Autodesk Fusion 360 part; units mm, degrees
(part 3 of 3)
  spline S28 degree 3 poles (32.7248, 18.541) (32.6316, 18.2641) (32.4511, 17.7282) (32.036, 17.3454) (31.8353, 17.1604) knots 0 0 0 0 0.086094 0.166606 0.166606 0.166606 0.166606
  spline S29 degree 3 poles (31.8353, 17.1604) (31.5951, 17.0173) (31.0851, 16.7134) (30.4908, 16.6845) (30.1764, 16.6692) knots 0 0 0 0 0.08261 0.175377 0.175377 0.175377 0.175377
  spline S30 degree 3 poles (30.1764, 16.6692) (29.7808, 16.6955) (29.0244, 16.7456) (28.4392, 17.2241) (28.16, 17.4523) knots 0 0 0 0 0.115653 0.221163 0.221163 0.221163 0.221163
  spline S31 degree 3 poles (28.16, 17.4523) (27.9431, 17.755) (27.4744, 18.4088) (27.4359, 19.2155) (27.4151, 19.6488) knots 0 0 0 0 0.109404 0.236358 0.236358 0.236358 0.236358
  spline S32 degree 3 poles (27.4151, 19.6488) (27.4356, 20.0964) (27.4735, 20.9274) (27.9489, 21.6059) (28.1682, 21.9189) knots 0 0 0 0 0.131235 0.243597 0.243597 0.243597 0.243597
  spline S33 degree 3 poles (28.1682, 21.9189) (28.4424, 22.1544) (29.0042, 22.6369) (29.7434, 22.6962) (30.1218, 22.7265) knots 0 0 0 0 0.105595 0.216319 0.216319 0.216319 0.216319
  spline S34 degree 3 poles (30.1218, 22.7265) (30.4889, 22.6964) (31.2082, 22.6372) (31.7537, 22.166) (32.0209, 21.9353) knots 0 0 0 0 0.10743 0.210533 0.210533 0.210533 0.210533
  spline S35 degree 3 poles (32.0209, 21.9353) (32.2354, 21.6284) (32.7008, 20.9627) (32.7377, 20.148) (32.7576, 19.7088) knots 0 0 0 0 0.110094 0.23884 0.23884 0.23884 0.23884
  spline S36 degree 3 poles (32.7576, 19.7088) (32.7572, 19.6724) (32.7564, 19.5851) (32.7537, 19.4978) (32.7521, 19.4469) knots 0 0 0 0 0.010915 0.0262 0.0262 0.0262 0.0262
  line L413 (32.7521, 19.4469) -> (28.4302, 19.4469)
  spline S37 degree 3 poles (28.4302, 19.4469) (28.4585, 19.1559) (28.5109, 18.619) (28.8261, 18.1837) (28.9704, 17.9844) knots 0 0 0 0 0.08586 0.158415 0.158415 0.158415 0.158415
  spline S38 degree 3 poles (34.5475, 5.4169) (34.5677, 5.3787) (34.6088, 5.3015) (34.6804, 5.2513) (34.7166, 5.2259) knots 0 0 0 0 0.012755 0.025838 0.025838 0.025838 0.025838
  spline S39 degree 3 poles (34.7166, 5.2259) (34.7635, 5.2052) (34.8701, 5.1584) (34.9868, 5.1562) (35.0522, 5.1549) knots 0 0 0 0 0.015217 0.034603 0.034603 0.034603 0.034603
  spline S40 degree 3 poles (35.0522, 5.1549) (35.1155, 5.1572) (35.2599, 5.1623) (35.403, 5.182) (35.4834, 5.1931) knots 0 0 0 0 0.018987 0.043304 0.043304 0.043304 0.043304
  line L414 (35.4834, 5.1931) -> (35.6252, 4.3254)
  spline S41 degree 3 poles (35.6252, 4.3254) (35.4947, 4.3) (35.2494, 4.2522) (34.9998, 4.2426) (34.8831, 4.2381) knots 0 0 0 0 0.039832 0.074826 0.074826 0.074826 0.074826
  spline S42 degree 3 poles (34.8831, 4.2381) (34.7224, 4.2412) (34.4348, 4.2468) (34.1703, 4.3581) (34.0536, 4.4073) knots 0 0 0 0 0.047664 0.085336 0.085336 0.085336 0.085336
  spline S43 degree 3 poles (34.0536, 4.4073) (33.9634, 4.4665) (33.7887, 4.5812) (33.6877, 4.7638) (33.6389, 4.8521) knots 0 0 0 0 0.031834 0.061632 0.061632 0.061632 0.061632
  spline S44 degree 3 poles (33.6389, 4.8521) (33.6044, 4.9941) (33.512, 5.3741) (33.5162, 5.7661) (33.5188, 6.0117) knots 0 0 0 0 0.043707 0.116961 0.116961 0.116961 0.116961
  line L415 (33.5188, 6.0117) -> (33.5188, 9.3459)
  line L416 (33.5188, 9.3459) -> (32.7985, 9.3459)
  line L417 (32.7985, 9.3459) -> (32.7985, 10.1099)
  line L418 (32.7985, 10.1099) -> (33.5188, 10.1099)
  line L419 (33.5188, 10.1099) -> (33.5188, 11.5451)
  line L420 (33.5188, 11.5451) -> (34.4956, 12.1345)
  line L421 (34.4956, 12.1345) -> (34.4956, 10.1099)
  line L422 (34.4956, 10.1099) -> (35.4834, 10.1099)
  line L423 (35.4834, 10.1099) -> (35.4834, 9.3459)
  line L424 (35.4834, 9.3459) -> (34.4956, 9.3459)
  line L425 (34.4956, 9.3459) -> (34.4956, 5.9571)
  spline S45 degree 3 poles (34.4956, 5.9571) (34.4942, 5.8414) (34.4919, 5.659) (34.5326, 5.4817) (34.5475, 5.4169) knots 0 0 0 0 0.03454 0.054433 0.054433 0.054433 0.054433
  spline S46 degree 3 poles (18.954, 8.5328) (18.9081, 8.3627) (18.8011, 7.9667) (18.7977, 7.5558) (18.7958, 7.3214) knots 0 0 0 0 0.052651 0.122613 0.122613 0.122613 0.122613
  line L426 (18.7958, 7.3214) -> (18.7958, 4.3145)
  line L427 (18.7958, 4.3145) -> (17.8135, 4.3145)
  line L428 (17.8135, 4.3145) -> (17.8135, 10.1099)
  line L429 (17.8135, 10.1099) -> (18.6921, 10.1099)
  line L430 (18.6921, 10.1099) -> (18.6921, 9.2968)
  spline S47 degree 3 poles (18.6921, 9.2968) (18.7912, 9.4321) (18.9909, 9.705) (19.2748, 9.8889) (19.4179, 9.9817) knots 0 0 0 0 0.049853 0.100536 0.100536 0.100536 0.100536
  spline S48 degree 3 poles (19.4179, 9.9817) (19.5766, 10.0572) (19.9028, 10.2126) (20.2638, 10.2313) (20.4493, 10.2409) knots 0 0 0 0 0.052187 0.107276 0.107276 0.107276 0.107276
  spline S49 degree 3 poles (20.4493, 10.2409) (20.6485, 10.2333) (21.0203, 10.2191) (21.3514, 10.0514) (21.5052, 9.9735) knots 0 0 0 0 0.058975 0.110073 0.110073 0.110073 0.110073
  spline S50 degree 3 poles (21.5052, 9.9735) (21.6327, 9.8747) (21.8901, 9.6752) (22.0205, 9.3766) (22.0864, 9.2259) knots 0 0 0 0 0.04756 0.096056 0.096056 0.096056 0.096056
  spline S51 degree 3 poles (22.0864, 9.2259) (22.3266, 9.5218) (22.7924, 10.0955) (23.5227, 10.1934) (23.8763, 10.2409) knots 0 0 0 0 0.1098 0.212838 0.212838 0.212838 0.212838
  spline S52 degree 3 poles (23.8763, 10.2409) (24.1404, 10.2274) (24.633, 10.2023) (25.0219, 9.9024) (25.2023, 9.7634) knots 0 0 0 0 0.07719 0.143952 0.143952 0.143952 0.143952
  spline S53 degree 3 poles (25.2023, 9.7634) (25.3372, 9.5677) (25.6403, 9.1278) (25.6569, 8.5908) (25.6662, 8.2927) knots 0 0 0 0 0.069911 0.157111 0.157111 0.157111 0.157111
  line L431 (25.6662, 8.2927) -> (25.6662, 4.3145)
  line L432 (25.6662, 4.3145) -> (24.6894, 4.3145)
  line L433 (24.6894, 4.3145) -> (24.6894, 7.9653)
  spline S54 degree 3 poles (24.6894, 7.9653) (24.6893, 8.1352) (24.6893, 8.4221) (24.6215, 8.7004) (24.5939, 8.8139) knots 0 0 0 0 0.050739 0.085655 0.085655 0.085655 0.085655
  spline S55 degree 3 poles (24.5939, 8.8139) (24.5548, 8.8965) (24.475, 9.0652) (24.3242, 9.1752) (24.2473, 9.2313) knots 0 0 0 0 0.026981 0.05503 0.05503 0.05503 0.05503
  spline S56 degree 3 poles (24.2473, 9.2313) (24.1582, 9.2775) (23.9735, 9.3731) (23.7656, 9.3839) (23.658, 9.3896) knots 0 0 0 0 0.029755 0.061652 0.061652 0.061652 0.061652
  spline S57 degree 3 poles (23.658, 9.3896) (23.4642, 9.3739) (23.0834, 9.3431) (22.788, 9.1016) (22.643, 8.983) knots 0 0 0 0 0.05685 0.111677 0.111677 0.111677 0.111677
  spline S58 degree 3 poles (22.643, 8.983) (22.5256, 8.8123) (22.2582, 8.4233) (22.246, 7.9482) (22.2392, 7.6815) knots 0 0 0 0 0.060926 0.138868 0.138868 0.138868 0.138868
  line L434 (22.2392, 7.6815) -> (22.2392, 4.3145)
  line L435 (22.2392, 4.3145) -> (21.2569, 4.3145)
  line L436 (21.2569, 4.3145) -> (21.2569, 8.0799)
  spline S59 degree 3 poles (21.2569, 8.0799) (21.253, 8.2752) (21.2462, 8.622) (21.0865, 8.9283) (21.0168, 9.0621) knots 0 0 0 0 0.057612 0.102327 0.102327 0.102327 0.102327
  spline S60 degree 3 poles (21.0168, 9.0621) (20.9172, 9.1575) (20.6993, 9.3661) (20.3958, 9.3813) (20.231, 9.3896) knots 0 0 0 0 0.04006 0.087699 0.087699 0.087699 0.087699
  spline S61 degree 3 poles (20.231, 9.3896) (20.0954, 9.3805) (19.8242, 9.3623) (19.5842, 9.235) (19.4643, 9.1713) knots 0 0 0 0 0.040276 0.080523 0.080523 0.080523 0.080523
  spline S62 degree 3 poles (19.4643, 9.1713) (19.3545, 9.0886) (19.1299, 8.9196) (19.0135, 8.6636) (18.954, 8.5328) knots 0 0 0 0 0.040543 0.082899 0.082899 0.082899 0.082899
  line L437 (15.5952, 33.335) -> (14.2855, 32.0581)
  line L438 (14.2855, 32.0581) -> (14.2855, 29.2859)
  line L439 (14.2855, 29.2859) -> (13.2269, 29.2859)
  line L440 (13.2269, 29.2859) -> (13.2269, 37.2859)
  line L441 (13.2269, 37.2859) -> (14.2855, 37.2859)
  line L442 (14.2855, 37.2859) -> (14.2855, 33.3186)
  line L443 (14.2855, 33.3186) -> (18.2583, 37.2859)
  line L444 (18.2583, 37.2859) -> (19.6935, 37.2859)
  line L445 (19.6935, 37.2859) -> (16.3374, 34.0444)
  line L446 (16.3374, 34.0444) -> (19.8408, 29.2859)
  line L447 (19.8408, 29.2859) -> (18.4438, 29.2859)
  line L448 (18.4438, 29.2859) -> (15.5952, 33.335)
  spline S63 degree 3 poles (28.0427, 30.4701) (28.2157, 30.322) (28.5649, 30.0232) (29.023, 29.9829) (29.2542, 29.9626) knots 0 0 0 0 0.066533 0.134307 0.134307 0.134307 0.134307
  spline S64 degree 3 poles (29.2542, 29.9626) (29.4253, 29.9727) (29.7563, 29.9922) (30.0396, 30.1636) (30.1764, 30.2463) knots 0 0 0 0 0.050568 0.097792 0.097792 0.097792 0.097792
  spline S65 degree 3 poles (30.1764, 30.2463) (30.2998, 30.3628) (30.5699, 30.6178) (30.7074, 30.964) (30.7821, 31.1522) knots 0 0 0 0 0.050293 0.110147 0.110147 0.110147 0.110147
  line L449 (30.7821, 31.1522) -> (31.7971, 31.0267)
  spline S66 degree 3 poles (31.7971, 31.0267) (31.7039, 30.7497) (31.5234, 30.2138) (31.1083, 29.831) (30.9076, 29.646) knots 0 0 0 0 0.086093 0.166606 0.166606 0.166606 0.166606
  spline S67 degree 3 poles (30.9076, 29.646) (30.6674, 29.5029) (30.1574, 29.1991) (29.5631, 29.1702) (29.2487, 29.1549) knots 0 0 0 0 0.082609 0.175376 0.175376 0.175376 0.175376
  spline S68 degree 3 poles (29.2487, 29.1549) (28.8532, 29.1811) (28.0967, 29.2313) (27.5115, 29.7097) (27.2323, 29.938) knots 0 0 0 0 0.115653 0.221163 0.221163 0.221163 0.221163
  spline S69 degree 3 poles (27.2323, 29.938) (27.0154, 30.2406) (26.5467, 30.8944) (26.5082, 31.7011) (26.4874, 32.1345) knots 0 0 0 0 0.109405 0.236358 0.236358 0.236358 0.236358
  spline S70 degree 3 poles (26.4874, 32.1345) (26.5079, 32.5821) (26.5458, 33.4131) (27.0212, 34.0916) (27.2405, 34.4046) knots 0 0 0 0 0.131235 0.243597 0.243597 0.243597 0.243597
  spline S71 degree 3 poles (27.2405, 34.4046) (27.5147, 34.6401) (28.0765, 35.1226) (28.8157, 35.1819) (29.1941, 35.2122) knots 0 0 0 0 0.105595 0.216319 0.216319 0.216319 0.216319
  spline S72 degree 3 poles (29.1941, 35.2122) (29.5612, 35.182) (30.2806, 35.1229) (30.826, 34.6517) (31.0932, 34.4209) knots 0 0 0 0 0.10743 0.210533 0.210533 0.210533 0.210533
  spline S73 degree 3 poles (31.0932, 34.4209) (31.3077, 34.1141) (31.7731, 33.4484) (31.81, 32.6336) (31.8299, 32.1945) knots 0 0 0 0 0.110094 0.238839 0.238839 0.238839 0.238839
  spline S74 degree 3 poles (31.8299, 32.1945) (31.8295, 32.1581) (31.8287, 32.0708) (31.826, 31.9835) (31.8244, 31.9325) knots 0 0 0 0 0.010915 0.0262 0.0262 0.0262 0.0262
  line L450 (31.8244, 31.9325) -> (27.5025, 31.9325)
  spline S75 degree 3 poles (27.5025, 31.9325) (27.5308, 31.6416) (27.5832, 31.1047) (27.8984, 30.6694) (28.0427, 30.4701) knots 0 0 0 0 0.08586 0.158415 0.158415 0.158415 0.158415
  line L451 (11.5652, 5.2586) -> (16.4765, 5.2586)
  line L452 (16.4765, 5.2586) -> (16.4765, 4.3145)
  line L453 (16.4765, 4.3145) -> (10.5065, 4.3145)
  line L454 (10.5065, 4.3145) -> (10.5065, 12.3145)
  line L455 (10.5065, 12.3145) -> (16.291, 12.3145)
  line L456 (16.291, 12.3145) -> (16.291, 11.3705)
  line L457 (16.291, 11.3705) -> (11.5652, 11.3705)
  line L458 (11.5652, 11.3705) -> (11.5652, 8.9203)
  line L459 (11.5652, 8.9203) -> (15.9909, 8.9203)
  line L460 (15.9909, 8.9203) -> (15.9909, 7.9817)
  line L461 (15.9909, 7.9817) -> (11.5652, 7.9817)
  line L462 (11.5652, 7.9817) -> (11.5652, 5.2586)
  spline S76 degree 3 poles (38.4411, 2.9012) (38.3557, 2.7537) (38.1975, 2.4803) (37.9533, 2.2809) (37.8408, 2.189) knots 0 0 0 0 0.050608 0.093822 0.093822 0.093822 0.093822
  spline S77 degree 3 poles (37.8408, 2.189) (37.7198, 2.123) (37.4683, 1.9857) (37.1818, 1.9705) (37.0332, 1.9626) knots 0 0 0 0 0.04081 0.084832 0.084832 0.084832 0.084832
  spline S78 degree 3 poles (37.0332, 1.9626) (36.9324, 1.9688) (36.7165, 1.9821) (36.5102, 2.0476) (36.4001, 2.0826) knots 0 0 0 0 0.030163 0.064648 0.064648 0.064648 0.064648
  line L463 (36.4001, 2.0826) -> (36.291, 3.0048)
  spline S79 degree 3 poles (36.291, 3.0048) (36.391, 2.9794) (36.5756, 2.9325) (36.7658, 2.9222) (36.8531, 2.9175) knots 0 0 0 0 0.030853 0.057001 0.057001 0.057001 0.057001
  spline S80 degree 3 poles (36.8531, 2.9175) (36.9528, 2.92) (37.1344, 2.9246) (37.3015, 2.9949) (37.3769, 3.0267) knots 0 0 0 0 0.029594 0.053932 0.053932 0.053932 0.053932
  spline S81 degree 3 poles (37.3769, 3.0267) (37.4397, 3.067) (37.5663, 3.1484) (37.6544, 3.2706) (37.6989, 3.3323) knots 0 0 0 0 0.022157 0.044743 0.044743 0.044743 0.044743
  spline S82 degree 3 poles (37.6989, 3.3323) (37.7407, 3.4172) (37.8571, 3.654) (37.9436, 3.9035) (37.999, 4.0635) knots 0 0 0 0 0.028377 0.079105 0.079105 0.079105 0.079105
  spline S83 degree 3 poles (37.999, 4.0635) (38.0107, 4.0972) (38.0387, 4.1777) (38.0688, 4.2573) (38.0864, 4.3036) knots 0 0 0 0 0.0107 0.02555 0.02555 0.02555 0.02555
  line L464 (38.0864, 4.3036) -> (35.8872, 10.1099)
  line L465 (35.8872, 10.1099) -> (36.9458, 10.1099)
  line L466 (36.9458, 10.1099) -> (38.1518, 6.7538)
  spline S84 degree 3 poles (38.1518, 6.7538) (38.2285, 6.5363) (38.3845, 6.0939) (38.5088, 5.6414) (38.572, 5.4114) knots 0 0 0 0 0.069157 0.140705 0.140705 0.140705 0.140705
  spline S85 degree 3 poles (38.572, 5.4114) (38.631, 5.6351) (38.7483, 6.0806) (38.9002, 6.5155) (38.9759, 6.732) knots 0 0 0 0 0.069376 0.138143 0.138143 0.138143 0.138143
  line L467 (38.9759, 6.732) -> (40.2146, 10.1099)
  line L468 (40.2146, 10.1099) -> (41.1969, 10.1099)
  line L469 (41.1969, 10.1099) -> (38.9922, 4.2163)
  spline S86 degree 3 poles (38.9922, 4.2163) (38.8921, 3.9454) (38.7272, 3.499) (38.5218, 3.0699) (38.4411, 2.9012) knots 0 0 0 0 0.086568 0.142661 0.142661 0.142661 0.142661
  line L470 (0, 41.4903) -> (2.5, 41.4903)
  line L471 (2.5, 41.4903) -> (2.5, 36.4903)
  line L472 (2.5, 36.4903) -> (0, 36.4903)
  line L473 (0, 36.4903) -> (0, 31.4903)
  line L474 (0, 31.4903) -> (2.5, 31.4903)
  line L475 (2.5, 31.4903) -> (2.5, 26.4903)
  line L476 (2.5, 26.4903) -> (0, 26.4903)
  line L477 (0, 26.4903) -> (0, 21.4903)
  line L478 (0, 21.4903) -> (2.5, 21.4903)
  line L479 (2.5, 21.4903) -> (2.5, 16.4903)
  line L480 (2.5, 16.4903) -> (0, 16.4903)
  line L481 (0, 16.4903) -> (0, 11.4903)
  line L482 (0, 11.4903) -> (2.5, 11.4903)
  line L483 (2.5, 11.4903) -> (2.5, 6.4903)
  line L484 (2.5, 6.4903) -> (0, 6.4903)
  line L485 (0, 6.4903) -> (0, -3.5097)
  line L486 (0, -3.5097) -> (2.5, -3.5097)
  line L487 (2.5, -3.5097) -> (2.5, -1.0097)
  line L488 (2.5, -1.0097) -> (7.5, -1.0097)
  line L489 (7.5, -1.0097) -> (7.5, -3.5097)
  line L490 (7.5, -3.5097) -> (12.5, -3.5097)
  line L491 (12.5, -3.5097) -> (12.5, -1.0097)
  line L492 (12.5, -1.0097) -> (17.5, -1.0097)
  line L493 (17.5, -1.0097) -> (17.5, -3.5097)
  line L494 (17.5, -3.5097) -> (22.5, -3.5097)
  line L495 (22.5, -3.5097) -> (22.5, -1.0097)
  line L496 (22.5, -1.0097) -> (27.5, -1.0097)
  line L497 (27.5, -1.0097) -> (27.5, -3.5097)
  line L498 (27.5, -3.5097) -> (32.5, -3.5097)
  line L499 (32.5, -3.5097) -> (32.5, -1.0097)
  line L500 (32.5, -1.0097) -> (37.5, -1.0097)
  line L501 (37.5, -1.0097) -> (37.5, -3.5097)
  line L502 (37.5, -3.5097) -> (42.5, -3.5097)
  line L503 (42.5, -3.5097) -> (42.5, -1.0097)
  line L504 (42.5, -1.0097) -> (47.5, -1.0097)
  line L505 (47.5, -1.0097) -> (47.5, -3.5097)
  line L506 (47.5, -3.5097) -> (50, -3.5097)
  line L507 (50, -3.5097) -> (50, 6.4903)
  line L508 (50, 6.4903) -> (47.5, 6.4903)
  line L509 (47.5, 6.4903) -> (47.5, 11.4903)
  line L510 (47.5, 11.4903) -> (50, 11.4903)
  line L511 (50, 11.4903) -> (50, 16.4903)
  line L512 (50, 16.4903) -> (47.5, 16.4903)
  line L513 (47.5, 16.4903) -> (47.5, 21.4903)
  line L514 (47.5, 21.4903) -> (50, 21.4903)
  line L515 (50, 21.4903) -> (50, 26.4903)
  line L516 (50, 26.4903) -> (47.5, 26.4903)
  line L517 (47.5, 26.4903) -> (47.5, 31.4903)
  line L518 (47.5, 31.4903) -> (50, 31.4903)
  line L519 (50, 31.4903) -> (50, 36.4903)
  line L520 (50, 36.4903) -> (47.5, 36.4903)
  line L521 (47.5, 36.4903) -> (47.5, 41.4903)
  line L522 (47.5, 41.4903) -> (50, 41.4903)
  line L523 (50, 41.4903) -> (50, 46.4903)
  line L524 (50, 46.4903) -> (47.3, 46.4903)
  line L525 (47.3, 46.4903) -> (47.3, 43.9903)
  line L526 (47.3, 43.9903) -> (42.7, 43.9903)
  line L527 (42.7, 43.9903) -> (42.7, 46.4903)
  line L528 (42.7, 46.4903) -> (37.3, 46.4903)
  line L529 (37.3, 46.4903) -> (37.3, 43.9903)
  line L530 (37.3, 43.9903) -> (32.7, 43.9903)
  line L531 (32.7, 43.9903) -> (32.7, 46.4903)
  line L532 (32.7, 46.4903) -> (27.3, 46.4903)
  line L533 (27.3, 46.4903) -> (27.3, 43.9903)
  line L534 (27.3, 43.9903) -> (22.7, 43.9903)
  line L535 (22.7, 43.9903) -> (22.7, 46.4903)
  line L536 (22.7, 46.4903) -> (17.3, 46.4903)
  line L537 (17.3, 46.4903) -> (17.3, 43.9903)
  line L538 (17.3, 43.9903) -> (12.7, 43.9903)
  line L539 (12.7, 43.9903) -> (12.7, 46.4903)
  line L540 (12.7, 46.4903) -> (7.3, 46.4903)
  line L541 (7.3, 46.4903) -> (7.3, 43.9903)
  line L542 (7.3, 43.9903) -> (2.7, 43.9903)
  line L543 (2.7, 43.9903) -> (2.7, 46.4903)
  line L544 (2.7, 46.4903) -> (0, 46.4903)
  line L545 (0, 46.4903) -> (0, 41.4903)
  spline S87 degree 3 poles (34.6539, 29.3623) (34.5306, 29.4347) (34.2897, 29.5762) (34.1036, 29.7844) (34.0127, 29.8862) knots 0 0 0 0 0.042587 0.083249 0.083249 0.083249 0.083249
  line L546 (34.0127, 29.8862) -> (34.0127, 27.0649)
  line L547 (34.0127, 27.0649) -> (33.0304, 27.0649)
  line L548 (33.0304, 27.0649) -> (33.0304, 35.0812)
  line L549 (33.0304, 35.0812) -> (33.9254, 35.0812)
  line L550 (33.9254, 35.0812) -> (33.9254, 34.3282)
  spline S88 degree 3 poles (33.9254, 34.3282) (34.031, 34.4644) (34.2329, 34.725) (34.5087, 34.9052) (34.6402, 34.9912) knots 0 0 0 0 0.051297 0.098108 0.098108 0.098108 0.098108
  spline S89 degree 3 poles (34.6402, 34.9912) (34.785, 35.0556) (35.092, 35.1923) (35.4283, 35.2053) (35.6061, 35.2122) knots 0 0 0 0 0.04708 0.099893 0.099893 0.099893 0.099893
  spline S90 degree 3 poles (35.6061, 35.2122) (35.8441, 35.1977) (36.3099, 35.1694) (36.7168, 34.9416) (36.9158, 34.8302) knots 0 0 0 0 0.0705 0.138 0.138 0.138 0.138
  spline S91 degree 3 poles (36.9158, 34.8302) (37.0946, 34.687) (37.4615, 34.3929) (37.6671, 33.9696) (37.7726, 33.7525) knots 0 0 0 0 0.06782 0.139223 0.139223 0.139223 0.139223
  spline S92 degree 3 poles (37.7726, 33.7525) (37.8569, 33.5117) (38.0299, 33.018) (38.051, 32.4951) (38.0618, 32.2272) knots 0 0 0 0 0.076077 0.15601 0.15601 0.15601 0.15601
  spline S93 degree 3 poles (38.0618, 32.2272) (38.0504, 31.9424) (38.0283, 31.3914) (37.8356, 30.875) (37.7426, 30.6256) knots 0 0 0 0 0.084892 0.164238 0.164238 0.164238 0.164238
  spline S94 degree 3 poles (37.7426, 30.6256) (37.6265, 30.4036) (37.3995, 29.9694) (37.0068, 29.677) (36.8149, 29.5342) knots 0 0 0 0 0.074084 0.14489 0.14489 0.14489 0.14489
  spline S95 degree 3 poles (36.8149, 29.5342) (36.6115, 29.4236) (36.2116, 29.2062) (35.758, 29.1718) (35.5352, 29.1549) knots 0 0 0 0 0.068591 0.134825 0.134825 0.134825 0.134825
  spline S96 degree 3 poles (35.5352, 29.1549) (35.3776, 29.1626) (35.0709, 29.1774) (34.7903, 29.3018) (34.6539, 29.3623) knots 0 0 0 0 0.046877 0.091234 0.091234 0.091234 0.091234
  line L551 (22.9786, 35.2122) -> (23.3457, 35.182)
  line L552 (23.3457, 35.182) -> (24.065, 35.1229)
  line L553 (24.065, 35.1229) -> (24.6105, 34.6517)
  line L554 (24.6105, 34.6517) -> (24.8776, 34.4209)
  line L555 (24.6921, 29.646) -> (24.4518, 29.5029)
  line L556 (24.4518, 29.5029) -> (23.9418, 29.1991)
  line L557 (23.9418, 29.1991) -> (23.3475, 29.1702)
  line L558 (23.3475, 29.1702) -> (23.0332, 29.1549)
  line L559 (27.2323, 29.938) -> (27.0154, 30.2406)
  line L560 (27.0154, 30.2406) -> (26.5467, 30.8944)
  line L561 (26.5467, 30.8944) -> (26.5082, 31.7011)
  line L562 (26.5082, 31.7011) -> (26.4874, 32.1345)
  line L563 (23.0332, 29.1549) -> (22.6376, 29.1811)
  line L564 (22.6376, 29.1811) -> (21.8812, 29.2313)
  line L565 (21.8812, 29.2313) -> (21.296, 29.7097)
  line L566 (21.296, 29.7097) -> (21.0168, 29.938)
  line L567 (25.6143, 32.1945) -> (25.614, 32.1581)
  line L568 (25.614, 32.1581) -> (25.6131, 32.0708)
  line L569 (25.6131, 32.0708) -> (25.6104, 31.9835)
  line L570 (25.6104, 31.9835) -> (25.6089, 31.9325)
  line L571 (24.8776, 34.4209) -> (25.0922, 34.1141)
  line L572 (25.0922, 34.1141) -> (25.5575, 33.4484)
  line L573 (25.5575, 33.4484) -> (25.5944, 32.6336)
  line L574 (25.5944, 32.6336) -> (25.6143, 32.1945)
  line L575 (21.0168, 29.938) -> (20.7998, 30.2406)
  line L576 (20.7998, 30.2406) -> (20.3312, 30.8944)
  line L577 (20.3312, 30.8944) -> (20.2926, 31.7011)
  line L578 (20.2926, 31.7011) -> (20.2719, 32.1345)
  line L579 (34.6402, 34.9912) -> (34.785, 35.0556)
  line L580 (34.785, 35.0556) -> (35.092, 35.1923)
  line L581 (35.092, 35.1923) -> (35.4283, 35.2053)
  line L582 (35.4283, 35.2053) -> (35.6061, 35.2122)
  line L583 (35.6252, 4.3254) -> (35.4947, 4.3)
  line L584 (35.4947, 4.3) -> (35.2494, 4.2522)
  line L585 (35.2494, 4.2522) -> (34.9998, 4.2426)
  line L586 (34.9998, 4.2426) -> (34.8831, 4.2381)
  line L587 (35.5352, 29.1549) -> (35.3776, 29.1626)
  line L588 (35.3776, 29.1626) -> (35.0709, 29.1774)
  line L589 (35.0709, 29.1774) -> (34.7903, 29.3018)
  line L590 (34.7903, 29.3018) -> (34.6539, 29.3623)
  line L591 (37.8408, 2.189) -> (37.7198, 2.123)
  line L592 (37.7198, 2.123) -> (37.4683, 1.9857)
  line L593 (37.4683, 1.9857) -> (37.1818, 1.9705)
  line L594 (37.1818, 1.9705) -> (37.0332, 1.9626)
  line L595 (37.7426, 30.6256) -> (37.6265, 30.4036)
  line L596 (37.6265, 30.4036) -> (37.3995, 29.9694)
  line L597 (37.3995, 29.9694) -> (37.0068, 29.677)
  line L598 (37.0068, 29.677) -> (36.8149, 29.5342)
  line L599 (34.7166, 5.2259) -> (34.7635, 5.2052)
  line L600 (34.7635, 5.2052) -> (34.8701, 5.1584)
  line L601 (34.8701, 5.1584) -> (34.9868, 5.1562)
  line L602 (34.9868, 5.1562) -> (35.0522, 5.1549)
  line L603 (36.8531, 2.9175) -> (36.9528, 2.92)
  line L604 (36.9528, 2.92) -> (37.1344, 2.9246)
  line L605 (37.1344, 2.9246) -> (37.3015, 2.9949)
  line L606 (37.3015, 2.9949) -> (37.3769, 3.0267)
  line L607 (30.1764, 16.6692) -> (29.7808, 16.6955)
  line L608 (29.7808, 16.6955) -> (29.0244, 16.7456)
  line L609 (29.0244, 16.7456) -> (28.4392, 17.2241)
  line L610 (28.4392, 17.2241) -> (28.16, 17.4523)
  line L611 (28.1682, 21.9189) -> (28.4424, 22.1544)
  line L612 (28.4424, 22.1544) -> (29.0042, 22.6369)
  line L613 (29.0042, 22.6369) -> (29.7434, 22.6962)
  line L614 (29.7434, 22.6962) -> (30.1218, 22.7265)
  line L615 (35.0522, 5.1549) -> (35.1155, 5.1572)
  line L616 (35.1155, 5.1572) -> (35.2599, 5.1623)
  line L617 (35.2599, 5.1623) -> (35.403, 5.182)
  line L618 (35.403, 5.182) -> (35.4834, 5.1931)
  line L619 (38.4411, 2.9012) -> (38.3557, 2.7537)
  line L620 (38.3557, 2.7537) -> (38.1975, 2.4803)
  line L621 (38.1975, 2.4803) -> (37.9533, 2.2809)
  line L622 (37.9533, 2.2809) -> (37.8408, 2.189)
  line L623 (31.8353, 17.1604) -> (31.5951, 17.0173)
  line L624 (31.5951, 17.0173) -> (31.0851, 16.7134)
  line L625 (31.0851, 16.7134) -> (30.4908, 16.6845)
  line L626 (30.4908, 16.6845) -> (30.1764, 16.6692)
  line L627 (36.291, 3.0048) -> (36.391, 2.9794)
  line L628 (36.391, 2.9794) -> (36.5756, 2.9325)
  line L629 (36.5756, 2.9325) -> (36.7658, 2.9222)
  line L630 (36.7658, 2.9222) -> (36.8531, 2.9175)
  line L631 (37.0332, 1.9626) -> (36.9324, 1.9688)
  line L632 (36.9324, 1.9688) -> (36.7165, 1.9821)
  line L633 (36.7165, 1.9821) -> (36.5102, 2.0476)
  line L634 (36.5102, 2.0476) -> (36.4001, 2.0826)
  line L635 (34.4956, 5.9571) -> (34.4942, 5.8414)
  line L636 (34.4942, 5.8414) -> (34.4919, 5.659)
  line L637 (34.4919, 5.659) -> (34.5326, 5.4817)
  line L638 (34.5326, 5.4817) -> (34.5475, 5.4169)
  line L639 (27.4151, 19.6488) -> (27.4356, 20.0964)
  line L640 (27.4356, 20.0964) -> (27.4735, 20.9274)
  line L641 (27.4735, 20.9274) -> (27.9489, 21.6059)
  line L642 (27.9489, 21.6059) -> (28.1682, 21.9189)
  line L643 (38.9922, 4.2163) -> (38.8921, 3.9454)
  line L644 (38.8921, 3.9454) -> (38.7272, 3.499)
  line L645 (38.7272, 3.499) -> (38.5218, 3.0699)
  line L646 (38.5218, 3.0699) -> (38.4411, 2.9012)
  line L647 (37.7726, 33.7525) -> (37.8569, 33.5117)
  line L648 (37.8569, 33.5117) -> (38.0299, 33.018)
  line L649 (38.0299, 33.018) -> (38.051, 32.4951)
  line L650 (38.051, 32.4951) -> (38.0618, 32.2272)
  line L651 (37.6989, 3.3323) -> (37.7407, 3.4172)
  line L652 (37.7407, 3.4172) -> (37.8571, 3.654)
  line L653 (37.8571, 3.654) -> (37.9436, 3.9035)
  line L654 (37.9436, 3.9035) -> (37.999, 4.0635)
  line L655 (32.7248, 18.541) -> (32.6316, 18.2641)
  line L656 (32.6316, 18.2641) -> (32.4511, 17.7282)
  line L657 (32.4511, 17.7282) -> (32.036, 17.3454)
  line L658 (32.036, 17.3454) -> (31.8353, 17.1604)
  line L659 (36.9158, 34.8302) -> (37.0946, 34.687)
  line L660 (37.0946, 34.687) -> (37.4615, 34.3929)
  line L661 (37.4615, 34.3929) -> (37.6671, 33.9696)
  line L662 (37.6671, 33.9696) -> (37.7726, 33.7525)
  line L663 (34.6539, 29.3623) -> (34.5306, 29.4347)
  line L664 (34.5306, 29.4347) -> (34.2897, 29.5762)
  line L665 (34.2897, 29.5762) -> (34.1036, 29.7844)
  line L666 (34.1036, 29.7844) -> (34.0127, 29.8862)
  line L667 (20.2719, 32.1345) -> (20.2923, 32.5821)
  line L668 (20.2923, 32.5821) -> (20.3302, 33.4131)
  line L669 (20.3302, 33.4131) -> (20.8057, 34.0916)
  line L670 (20.8057, 34.0916) -> (21.025, 34.4046)
  line L671 (21.2869, 31.9325) -> (21.3153, 31.6416)
  line L672 (21.3153, 31.6416) -> (21.3677, 31.1047)
  line L673 (21.3677, 31.1047) -> (21.6828, 30.6694)
  line L674 (21.6828, 30.6694) -> (21.8271, 30.4701)
  line L675 (25.5816, 31.0267) -> (25.4883, 30.7497)
  line L676 (25.4883, 30.7497) -> (25.3079, 30.2138)
  line L677 (25.3079, 30.2138) -> (24.8927, 29.831)
  line L678 (24.8927, 29.831) -> (24.6921, 29.646)
  line L679 (23.9608, 30.2463) -> (24.0842, 30.3628)
  line L680 (24.0842, 30.3628) -> (24.3544, 30.6178)
  line L681 (24.3544, 30.6178) -> (24.4919, 30.964)
  line L682 (24.4919, 30.964) -> (24.5666, 31.1522)
  line L683 (23.0386, 29.9626) -> (23.2097, 29.9727)
  line L684 (23.2097, 29.9727) -> (23.5407, 29.9922)
  line L685 (23.5407, 29.9922) -> (23.824, 30.1636)
  line L686 (23.824, 30.1636) -> (23.9608, 30.2463)
  line L687 (26.4874, 32.1345) -> (26.5079, 32.5821)
  line L688 (26.5079, 32.5821) -> (26.5458, 33.4131)
  line L689 (26.5458, 33.4131) -> (27.0212, 34.0916)
  line L690 (27.0212, 34.0916) -> (27.2405, 34.4046)
  line L691 (21.8271, 30.4701) -> (22.0001, 30.322)
  line L692 (22.0001, 30.322) -> (22.3494, 30.0232)
  line L693 (22.3494, 30.0232) -> (22.8074, 29.9829)
  line L694 (22.8074, 29.9829) -> (23.0386, 29.9626)
  line L695 (21.025, 34.4046) -> (21.2992, 34.6401)
  line L696 (21.2992, 34.6401) -> (21.8609, 35.1226)
  line L697 (21.8609, 35.1226) -> (22.6002, 35.1819)
  line L698 (22.6002, 35.1819) -> (22.9786, 35.2122)
  line L699 (31.0932, 34.4209) -> (31.3077, 34.1141)
  line L700 (31.3077, 34.1141) -> (31.7731, 33.4484)
  line L701 (31.7731, 33.4484) -> (31.81, 32.6336)
  line L702 (31.81, 32.6336) -> (31.8299, 32.1945)
  line L703 (31.0086, 9.8589) -> (31.1873, 9.7156)
  line L704 (31.1873, 9.7156) -> (31.5543, 9.4215)
  line L705 (31.5543, 9.4215) -> (31.7599, 8.9982)
  line L706 (31.7599, 8.9982) -> (31.8653, 8.7811)
  line L707 (30.9076, 29.646) -> (30.6674, 29.5029)
  line L708 (30.6674, 29.5029) -> (30.1574, 29.1991)
  line L709 (30.1574, 29.1991) -> (29.5631, 29.1702)
  line L710 (29.5631, 29.1702) -> (29.2487, 29.1549)
  line L711 (31.8653, 8.7811) -> (31.9497, 8.5404)
  line L712 (31.9497, 8.5404) -> (32.1226, 8.0467)
  line L713 (32.1226, 8.0467) -> (32.1438, 7.5238)
  line L714 (32.1438, 7.5238) -> (32.1546, 7.2559)
  line L715 (28.0427, 30.4701) -> (28.2157, 30.322)
  line L716 (28.2157, 30.322) -> (28.5649, 30.0232)
  line L717 (28.5649, 30.0232) -> (29.023, 29.9829)
  line L718 (29.023, 29.9829) -> (29.2542, 29.9626)
  line L719 (23.658, 9.3896) -> (23.4642, 9.3739)
  line L720 (23.4642, 9.3739) -> (23.0834, 9.3431)
  line L721 (23.0834, 9.3431) -> (22.788, 9.1016)
  line L722 (22.788, 9.1016) -> (22.643, 8.983)
  line L723 (32.7576, 19.7088) -> (32.7572, 19.6724)
  line L724 (32.7572, 19.6724) -> (32.7564, 19.5851)
  line L725 (32.7564, 19.5851) -> (32.7537, 19.4978)
  line L726 (32.7537, 19.4978) -> (32.7521, 19.4469)
  line L727 (27.5025, 31.9325) -> (27.5308, 31.6416)
  line L728 (27.5308, 31.6416) -> (27.5832, 31.1047)
  line L729 (27.5832, 31.1047) -> (27.8984, 30.6694)
  line L730 (27.8984, 30.6694) -> (28.0427, 30.4701)
  line L731 (18.6921, 9.2968) -> (18.7912, 9.4321)
  line L732 (18.7912, 9.4321) -> (18.9909, 9.705)
  line L733 (18.9909, 9.705) -> (19.2748, 9.8889)
  line L734 (19.2748, 9.8889) -> (19.4179, 9.9817)
  line L735 (28.16, 17.4523) -> (27.9431, 17.755)
  line L736 (27.9431, 17.755) -> (27.4744, 18.4088)
  line L737 (27.4744, 18.4088) -> (27.4359, 19.2155)
  line L738 (27.4359, 19.2155) -> (27.4151, 19.6488)
  line L739 (30.1764, 30.2463) -> (30.2998, 30.3628)
  line L740 (30.2998, 30.3628) -> (30.5699, 30.6178)
  line L741 (30.5699, 30.6178) -> (30.7074, 30.964)
  line L742 (30.7074, 30.964) -> (30.7821, 31.1522)
  line L743 (33.6389, 4.8521) -> (33.6044, 4.9941)
  line L744 (33.6044, 4.9941) -> (33.512, 5.3741)
  line L745 (33.512, 5.3741) -> (33.5162, 5.7661)
  line L746 (33.5162, 5.7661) -> (33.5188, 6.0117)
  line L747 (22.0864, 9.2259) -> (22.3266, 9.5218)
  line L748 (22.3266, 9.5218) -> (22.7924, 10.0955)
  line L749 (22.7924, 10.0955) -> (23.5227, 10.1934)
  line L750 (23.5227, 10.1934) -> (23.8763, 10.2409)
  line L751 (29.628, 4.1836) -> (29.4704, 4.1912)
  line L752 (29.4704, 4.1912) -> (29.1636, 4.2061)
  line L753 (29.1636, 4.2061) -> (28.8831, 4.3305)
  line L754 (28.8831, 4.3305) -> (28.7467, 4.3909)
  line L755 (29.6989, 10.2409) -> (29.9369, 10.2264)
  line L756 (29.9369, 10.2264) -> (30.4026, 10.198)
  line L757 (30.4026, 10.198) -> (30.8096, 9.9703)
  line L758 (30.8096, 9.9703) -> (31.0086, 9.8589)
  line L759 (22.3947, 17.9516) -> (22.4524, 18.1314)
  line L760 (22.4524, 18.1314) -> (22.5902, 18.5603)
  line L761 (22.5902, 18.5603) -> (22.7358, 18.9865)
  line L762 (22.7358, 18.9865) -> (22.8203, 19.234)
  line L763 (28.733, 10.0199) -> (28.8777, 10.0843)
  line L764 (28.8777, 10.0843) -> (29.1848, 10.2209)
  line L765 (29.1848, 10.2209) -> (29.5211, 10.234)
  line L766 (29.5211, 10.234) -> (29.6989, 10.2409)
  line L767 (29.1941, 35.2122) -> (29.5612, 35.182)
  line L768 (29.5612, 35.182) -> (30.2806, 35.1229)
  line L769 (30.2806, 35.1229) -> (30.826, 34.6517)
  line L770 (30.826, 34.6517) -> (31.0932, 34.4209)
  line L771 (19.4643, 9.1713) -> (19.3545, 9.0886)
  line L772 (19.3545, 9.0886) -> (19.1299, 8.9196)
  line L773 (19.1299, 8.9196) -> (19.0135, 8.6636)
  line L774 (19.0135, 8.6636) -> (18.954, 8.5328)
  line L775 (38.1518, 6.7538) -> (38.2285, 6.5363)
  line L776 (38.2285, 6.5363) -> (38.3845, 6.0939)
  line L777 (38.3845, 6.0939) -> (38.5088, 5.6414)
  line L778 (38.5088, 5.6414) -> (38.572, 5.4114)
  line L779 (28.7467, 4.3909) -> (28.6234, 4.4633)
  line L780 (28.6234, 4.4633) -> (28.3825, 4.6049)
  line L781 (28.3825, 4.6049) -> (28.1964, 4.8131)
  line L782 (28.1964, 4.8131) -> (28.1055, 4.9148)
  line L783 (32.0209, 21.9353) -> (32.2354, 21.6284)
  line L784 (32.2354, 21.6284) -> (32.7008, 20.9627)
  line L785 (32.7008, 20.9627) -> (32.7377, 20.148)
  line L786 (32.7377, 20.148) -> (32.7576, 19.7088)
  line L787 (20.4493, 10.2409) -> (20.6485, 10.2333)
  line L788 (20.6485, 10.2333) -> (21.0203, 10.2191)
  line L789 (21.0203, 10.2191) -> (21.3514, 10.0514)
  line L790 (21.3514, 10.0514) -> (21.5052, 9.9735)
  line L791 (31.8299, 32.1945) -> (31.8295, 32.1581)
  line L792 (31.8295, 32.1581) -> (31.8287, 32.0708)
  line L793 (31.8287, 32.0708) -> (31.826, 31.9835)
  line L794 (31.826, 31.9835) -> (31.8244, 31.9325)
  line L795 (18.954, 8.5328) -> (18.9081, 8.3627)
  line L796 (18.9081, 8.3627) -> (18.8011, 7.9667)
  line L797 (18.8011, 7.9667) -> (18.7977, 7.5558)
  line L798 (18.7977, 7.5558) -> (18.7958, 7.3214)
  line L799 (34.5475, 5.4169) -> (34.5677, 5.3787)
  line L800 (34.5677, 5.3787) -> (34.6088, 5.3015)
  line L801 (34.6088, 5.3015) -> (34.6804, 5.2513)
  line L802 (34.6804, 5.2513) -> (34.7166, 5.2259)
  line L803 (28.4302, 19.4469) -> (28.4585, 19.1559)
  line L804 (28.4585, 19.1559) -> (28.5109, 18.619)
  line L805 (28.5109, 18.619) -> (28.8261, 18.1837)
  line L806 (28.8261, 18.1837) -> (28.9704, 17.9844)
  line L807 (31.8353, 5.6542) -> (31.7193, 5.4322)
  line L808 (31.7193, 5.4322) -> (31.4922, 4.9981)
  line L809 (31.4922, 4.9981) -> (31.0995, 4.7057)
  line L810 (31.0995, 4.7057) -> (30.9076, 4.5628)
  line L811 (33.9254, 34.3282) -> (34.031, 34.4644)
  line L812 (34.031, 34.4644) -> (34.2329, 34.725)
  line L813 (34.2329, 34.725) -> (34.5087, 34.9052)
  line L814 (34.5087, 34.9052) -> (34.6402, 34.9912)
  line L815 (32.1546, 7.2559) -> (32.1432, 6.9711)
  line L816 (32.1432, 6.9711) -> (32.1211, 6.4201)
  line L817 (32.1211, 6.4201) -> (31.9284, 5.9037)
  line L818 (31.9284, 5.9037) -> (31.8353, 5.6542)
  line L819 (38.0618, 32.2272) -> (38.0504, 31.9424)
  line L820 (38.0504, 31.9424) -> (38.0283, 31.3914)
  line L821 (38.0283, 31.3914) -> (37.8356, 30.875)
  line L822 (37.8356, 30.875) -> (37.7426, 30.6256)
  line L823 (29.2542, 29.9626) -> (29.4253, 29.9727)
  line L824 (29.4253, 29.9727) -> (29.7563, 29.9922)
  line L825 (29.7563, 29.9922) -> (30.0396, 30.1636)
  line L826 (30.0396, 30.1636) -> (30.1764, 30.2463)
  line L827 (31.1041, 17.7606) -> (31.2275, 17.8771)
  line L828 (31.2275, 17.8771) -> (31.4976, 18.1321)
  line L829 (31.4976, 18.1321) -> (31.6351, 18.4784)
  line L830 (31.6351, 18.4784) -> (31.7098, 18.6665)
  line L831 (38.572, 5.4114) -> (38.631, 5.6351)
  line L832 (38.631, 5.6351) -> (38.7483, 6.0806)
  line L833 (38.7483, 6.0806) -> (38.9002, 6.5155)
  line L834 (38.9002, 6.5155) -> (38.9759, 6.732)
  line L835 (35.6061, 35.2122) -> (35.8441, 35.1977)
  line L836 (35.8441, 35.1977) -> (36.3099, 35.1694)
  line L837 (36.3099, 35.1694) -> (36.7168, 34.9416)
  line L838 (36.7168, 34.9416) -> (36.9158, 34.8302)
  line L839 (30.1819, 17.4769) -> (30.353, 17.487)
  line L840 (30.353, 17.487) -> (30.684, 17.5066)
  line L841 (30.684, 17.5066) -> (30.9673, 17.6779)
  line L842 (30.9673, 17.6779) -> (31.1041, 17.7606)
  line L843 (22.0127, 19.1358) -> (22.0889, 18.9055)
  line L844 (22.0889, 18.9055) -> (22.2192, 18.5117)
  line L845 (22.2192, 18.5117) -> (22.3432, 18.1159)
  line L846 (22.3432, 18.1159) -> (22.3947, 17.9516)
  line L847 (36.8149, 29.5342) -> (36.6115, 29.4236)
  line L848 (36.6115, 29.4236) -> (36.2116, 29.2062)
  line L849 (36.2116, 29.2062) -> (35.758, 29.1718)
  line L850 (35.758, 29.1718) -> (35.5352, 29.1549)
  line L851 (28.9704, 17.9844) -> (29.1434, 17.8364)
  line L852 (29.1434, 17.8364) -> (29.4926, 17.5376)
  line L853 (29.4926, 17.5376) -> (29.9507, 17.4972)
  line L854 (29.9507, 17.4972) -> (30.1819, 17.4769)
  line L855 (28.0181, 9.3568) -> (28.1237, 9.4931)
  line L856 (28.1237, 9.4931) -> (28.3257, 9.7536)
  line L857 (28.3257, 9.7536) -> (28.6015, 9.9339)
  line L858 (28.6015, 9.9339) -> (28.733, 10.0199)
  line L859 (31.7971, 31.0267) -> (31.7039, 30.7497)
  line L860 (31.7039, 30.7497) -> (31.5234, 30.2138)
  line L861 (31.5234, 30.2138) -> (31.1083, 29.831)
  line L862 (31.1083, 29.831) -> (30.9076, 29.646)
  line L863 (37.999, 4.0635) -> (38.0107, 4.0972)
  line L864 (38.0107, 4.0972) -> (38.0387, 4.1777)
  line L865 (38.0387, 4.1777) -> (38.0688, 4.2573)
  line L866 (38.0688, 4.2573) -> (38.0864, 4.3036)
  line L867 (30.1218, 22.7265) -> (30.4889, 22.6964)
  line L868 (30.4889, 22.6964) -> (31.2082, 22.6372)
  line L869 (31.2082, 22.6372) -> (31.7537, 22.166)
  line L870 (31.7537, 22.166) -> (32.0209, 21.9353)
  line L871 (37.3769, 3.0267) -> (37.4397, 3.067)
  line L872 (37.4397, 3.067) -> (37.5663, 3.1484)
  line L873 (37.5663, 3.1484) -> (37.6544, 3.2706)
  line L874 (37.6544, 3.2706) -> (37.6989, 3.3323)
  line L875 (21.5052, 9.9735) -> (21.6327, 9.8747)
  line L876 (21.6327, 9.8747) -> (21.8901, 9.6752)
  line L877 (21.8901, 9.6752) -> (22.0205, 9.3766)
  line L878 (22.0205, 9.3766) -> (22.0864, 9.2259)
  line L879 (21.0168, 9.0621) -> (20.9172, 9.1575)
  line L880 (20.9172, 9.1575) -> (20.6993, 9.3661)
  line L881 (20.6993, 9.3661) -> (20.3958, 9.3813)
  line L882 (20.3958, 9.3813) -> (20.231, 9.3896)
  line L883 (19.4179, 9.9817) -> (19.5766, 10.0572)
  line L884 (19.5766, 10.0572) -> (19.9028, 10.2126)
  line L885 (19.9028, 10.2126) -> (20.2638, 10.2313)
  line L886 (20.2638, 10.2313) -> (20.4493, 10.2409)
  line L887 (22.643, 8.983) -> (22.5256, 8.8123)
  line L888 (22.5256, 8.8123) -> (22.2582, 8.4233)
  line L889 (22.2582, 8.4233) -> (22.246, 7.9482)
  line L890 (22.246, 7.9482) -> (22.2392, 7.6815)
  line L891 (20.231, 9.3896) -> (20.0954, 9.3805)
  line L892 (20.0954, 9.3805) -> (19.8242, 9.3623)
  line L893 (19.8242, 9.3623) -> (19.5842, 9.235)
  line L894 (19.5842, 9.235) -> (19.4643, 9.1713)
  line L895 (34.8831, 4.2381) -> (34.7224, 4.2412)
  line L896 (34.7224, 4.2412) -> (34.4348, 4.2468)
  line L897 (34.4348, 4.2468) -> (34.1703, 4.3581)
  line L898 (34.1703, 4.3581) -> (34.0536, 4.4073)
  line L899 (24.2473, 9.2313) -> (24.1582, 9.2775)
  line L900 (24.1582, 9.2775) -> (23.9735, 9.3731)
  line L901 (23.9735, 9.3731) -> (23.7656, 9.3839)
  line L902 (23.7656, 9.3839) -> (23.658, 9.3896)
  line L903 (23.8763, 10.2409) -> (24.1404, 10.2274)
  line L904 (24.1404, 10.2274) -> (24.633, 10.2023)
  line L905 (24.633, 10.2023) -> (25.0219, 9.9024)
  line L906 (25.0219, 9.9024) -> (25.2023, 9.7634)
  line L907 (21.2569, 8.0799) -> (21.253, 8.2752)
  line L908 (21.253, 8.2752) -> (21.2462, 8.622)
  line L909 (21.2462, 8.622) -> (21.0865, 8.9283)
  line L910 (21.0865, 8.9283) -> (21.0168, 9.0621)
  line L911 (29.2487, 29.1549) -> (28.8532, 29.1811)
  line L912 (28.8532, 29.1811) -> (28.0967, 29.2313)
  line L913 (28.0967, 29.2313) -> (27.5115, 29.7097)
  line L914 (27.5115, 29.7097) -> (27.2323, 29.938)
  line L915 (25.2023, 9.7634) -> (25.3372, 9.5677)
  line L916 (25.3372, 9.5677) -> (25.6403, 9.1278)
  line L917 (25.6403, 9.1278) -> (25.6569, 8.5908)
  line L918 (25.6569, 8.5908) -> (25.6662, 8.2927)
  line L919 (34.0536, 4.4073) -> (33.9634, 4.4665)
  line L920 (33.9634, 4.4665) -> (33.7887, 4.5812)
  line L921 (33.7887, 4.5812) -> (33.6877, 4.7638)
  line L922 (33.6877, 4.7638) -> (33.6389, 4.8521)
  line L923 (27.2405, 34.4046) -> (27.5147, 34.6401)
  line L924 (27.5147, 34.6401) -> (28.0765, 35.1226)
  line L925 (28.0765, 35.1226) -> (28.8157, 35.1819)
  line L926 (28.8157, 35.1819) -> (29.1941, 35.2122)
  line L927 (30.9076, 4.5628) -> (30.7042, 4.4522)
  line L928 (30.7042, 4.4522) -> (30.3044, 4.2348)
  line L929 (30.3044, 4.2348) -> (29.8508, 4.2004)
  line L930 (29.8508, 4.2004) -> (29.628, 4.1836)
  line L931 (24.6894, 7.9653) -> (24.6893, 8.1352)
  line L932 (24.6893, 8.1352) -> (24.6893, 8.4221)
  line L933 (24.6893, 8.4221) -> (24.6215, 8.7004)
  line L934 (24.6215, 8.7004) -> (24.5939, 8.8139)
  line L935 (24.5939, 8.8139) -> (24.5548, 8.8965)
  line L936 (24.5548, 8.8965) -> (24.475, 9.0652)
  line L937 (24.475, 9.0652) -> (24.3242, 9.1752)
  line L938 (24.3242, 9.1752) -> (24.2473, 9.2313)
copy_body "Body->Comp2" [suppressed] in component "Component'"
component "Component" placed x (1, 0, 0) y (0, 0, 1) z (0, -1, 0) at (0, 46.4903, 23.4903)
component "Component''" placed x (0, 0, 1) y (0, 1, 0) z (-1, 0, 0) at (-8.993, 54.1484, 19.6977)
component "Component''" placed x (0, 0, -1) y (0, 1, 0) z (1, 0, 0) at (68.7168, 48.3116, 26.2404)
component "Component'''" placed x (1, 0, 0) y (0, 1, 0) z (0, 0, 1) at (0, 60, 2.5)
component "Component'''" placed x (1, 0, 0) y (0, 1, 0) z (0, 0, 1) at (70, 0, 50)
hidden bodies 6
equation "Length = 50 mm"
equation "Width = 50 mm"
equation "d5 = Length"
equation "d6 = Width"
equation "jl = 5 mm"
equation "jw = 2.5 mm"
equation "d9 = jw"
equation "d10 = jl"
equation "d14 = ( Length / jl ) * 1 mm"
equation "d19 = jw"
equation "d20 = jl"
equation "d21 = jl"
equation "d24 = ( -Width / jl ) * 1 mm"
equation "kurv = 0.4 mm"
equation "d29 = Length"
equation "d30 = Width"
equation "d31 = jw"
equation "d32 = jl + kurv"
equation "d33 = jl + kurv"
equation "d36 = ( -Length / jl ) * 1 mm"
equation "d38 = jw"
equation "d39 = jl"
equation "d40 = jw"
equation "d71 = Length - jw"
equation "d72 = Width"
equation "d77 = kurv / 2"
equation "d79 = kurv / 2"
equation "d81 = kurv / 2"
equation "d83 = kurv / 2"
equation "d85 = kurv / 2"
equation "d87 = kurv / 2"
equation "d89 = kurv / 2"
equation "d91 = kurv / 2"
equation "d93 = kurv / 2"
equation "d95 = kurv / 2"
equation "d97 = kurv / 2"
equation "d99 = kurv / 2"
equation "d101 = kurv / 2"
equation "d103 = kurv / 2"
equation "d105 = kurv / 2"
equation "d107 = kurv / 2"
equation "d109 = kurv / 2"
equation "d111 = kurv / 2"
equation "d113 = kurv / 2"
equation "d115 = kurv / 2"
equation "d117 = kurv / 2"
equation "d119 = kurv / 2"
equation "d121 = kurv / 2"
equation "d123 = kurv / 2"
equation "d125 = kurv / 2"
equation "d127 = kurv / 2"
